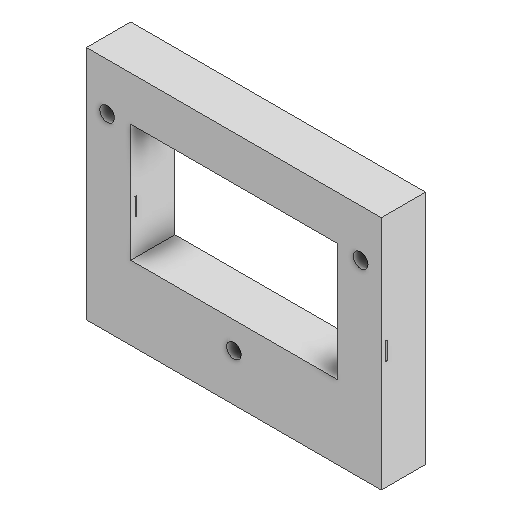
# Autodesk Inventor part: płytka_prowadzaca_rysik
Saved by Autodesk Inventor 2025.1 (Build 291241000, 241)
## iProperties
Created: 2025-04-08
Part Number: płytka_prowadzaca_rysik
Material: Ogólny
Document SubType Name: Modeling
Designer: Maciej
Density: 1 g/cm^3
Appearance: Domyślna
Author: Maciej
Autodesk Inventor part; units mm, degrees
ref_plane "YZ Plane" through (0, 0, 0) normal (1, 0, 0) x (0, 1, 0)
ref_plane "XZ Plane" through (0, 0, 0) normal (0, 1, 0) x (-1, 0, 0)
ref_plane "XY Plane" through (0, 0, 0) normal (0, 0, 1) x (1, 0, 0)
sketch "Szkic5" plane through (0, 0, 0) normal (0, 0, 1) x (1, 0, 0)
  line L0 (-50, -40) -> (50, -40)
  line L1 (50, -40) -> (50, 40)
  line L2 (50, 40) -> (-50, 40)
  line L3 (-50, 40) -> (-50, -40)
  line L4 (-50, -40) -> (50, 40) construction
  line L5 (50, -40) -> (-50, 40) construction
  line L6 (-35, -25) -> (35, -25)
  line L7 (35, -25) -> (35, 25)
  line L8 (35, 25) -> (-35, 25)
  line L9 (-35, 25) -> (-35, -25)
  line L10 (-35, -25) -> (35, 25) construction
  line L11 (35, -25) -> (-35, 25) construction
  point P0 (0, 0)
  dimension "d27" = 100
  dimension "d28" = 80
  dimension "d29" = 70
  dimension "d30" = 50
  constraints: 24 end point, 4 midpoint, 4 parallel, 2 horizontal, 2 perpendicular
  measures "d27" distance of L2.end L1.end
  measures "d28" distance of L1.end L0.end
  measures "d29" distance of L8.end L7.end
  measures "d30" distance of L7.end L6.end
extrude "Wyciągnięcie proste4" add sketch "Szkic5" against normal blind 13
sketch "Szkic6" plane through (0, 0, 0) normal (0, 0, 1) x (1, 0, 0)
  line L0 (-50, -40) -> (50, -40)
  line L1 (50, -40) -> (50, 40)
  line L2 (50, 40) -> (-50, 40)
  line L3 (-50, 40) -> (-50, -40)
  line L4 (-50, -40) -> (50, 40) construction
  line L5 (50, -40) -> (-50, 40) construction
  line L6 (35, -25) -> (35, 25) projected
  line L7 (-35, -25) -> (35, -25)
  line L8 (35, -25) -> (35, 25)
  line L9 (35, 25) -> (-35, 25)
  line L10 (-35, 25) -> (-35, -25)
  line L11 (-35, -25) -> (35, 25) construction
  line L12 (35, -25) -> (-35, 25) construction
  point P0 (0, 0)
  constraints: 24 end point, 4 midpoint, 4 parallel, 2 horizontal, 2 perpendicular
extrude "Wyciągnięcie proste5" add sketch "Szkic6" along normal blind 2
sketch "Szkic7" plane through (50, -40, -13) normal (1, 0, 0) x (0, 0, -1)
  line L0 (-13, 37) -> (-13.5, 37)
  line L1 (-13.5, 37) -> (-13.5, 43)
  line L2 (-13.5, 43) -> (-13, 43)
  line L3 (-13, 43) -> (-13, 37)
  line L4 (-13, 37) -> (-13.5, 43) construction
  line L5 (-13.5, 37) -> (-13, 43) construction
  line L6 (-15, 0) -> (-15, 80) projected
  line L7 (0, 80) -> (-15, 80) projected
  point P0 (-13, 40)
  point P1 (-13.25, 40)
  dimension "d35" = 0.5
  dimension "d36" = 6
  dimension "d37" = 1.5
  dimension "d38" = 40
  constraints: 12 end point, 2 midpoint, 2 parallel, 1 horizontal, 1 perpendicular
  measures "d35" distance of L1.end L2.end
  measures "d36" distance of L0.end L1.end
  measures "d37" distance between parallel lines of L6 L1
  measures "d38" distance from line of L7 point (-13.25, 40)
extrude "Wyciągnięcie proste6" cut sketch "Szkic7" against normal through all
sketch "Szkic8" plane through (-35, -25, -13) normal (0, 1, 0) x (1, 0, 0)
  line L0 (70, -15) -> (0, -15) projected
  line L1 (0, 0) -> (70, 0) projected
  line L2 (0, -15) -> (0, 0)
  line L3 (0, 0) -> (70, 0)
  line L4 (70, 0) -> (70, -15)
  line L5 (70, -15) -> (0, -15)
  point P0 (35, -13)
  constraints: 8 end point, 2 perpendicular, 1 collinear, 1 vertical
extrude "Wyciągnięcie proste7" add sketch "Szkic8" along normal blind 10
sketch "Szkic9" plane through (0, 0, 2) normal (0, 0, 1) x (1, 0, 0)
  line L0 (50, 40) -> (-50, 40) projected
  line L1 (-50, 40) -> (-50, -40) projected
  line L2 (50, -40) -> (50, 40) projected
  line L3 (-50, -40) -> (50, -40) projected
  point P0 (0, 0)
  point P1 (-43, 24)
  point P2 (43, 24)
  point P3 (0, -24.05)
  dimension "d43" = 16
  dimension "d44" = 16
  dimension "d45" = 7
  dimension "d46" = 7
  dimension "d54" = 15.95
  dimension "d55" = 50
  measures "d43" distance from line of L0 point (-43, 24)
  measures "d44" distance from line of L0 point (43, 24)
  measures "d45" distance from line of L1 point (-43, 24)
  measures "d46" distance from line of L2 point (43, 24)
  measures "d54" distance from line of L3 point (0, -24.05)
  measures "d55" distance from line of L1 point (0, -24.05)
hole "Otwór2" at (-43, 24, 2) at (43, 24, 2) at (0, -24.05, 2) direction (0, 0, -1) diameter 5 depth 15 tip angle 118 clearance for "Śruba ze łbem płaskim obrobiona" size "M4" standard "ANSI Profil metryczny M"
equation "\"d44\" = d43"
equation "\"d46\" = d45"
